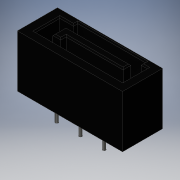
# Autodesk Inventor part: SATA_Conn_TH
Saved by Autodesk Inventor 2016 (Build 200138000, 138)
## iProperties
Created: 2017-03-04
Part Number: SATA_Conn_TH
Material: Generic
Document SubType Name: Modeling
Designer: jfixelle
Density: 1 g/cm^3
Appearance: Smooth - Black
Author: jfixelle
Autodesk Inventor part; units mm, degrees
ref_plane "YZ Plane" through (0, 0, 0) normal (1, 0, 0) x (0, 1, 0)
ref_plane "XZ Plane" through (0, 0, 0) normal (0, 1, 0) x (-1, 0, 0)
ref_plane "XY Plane" through (0, 0, 0) normal (0, 0, 1) x (1, 0, 0)
sketch "Sketch1" plane through (0, 0, 0) normal (0, 1, 0) x (-1, 0, 0)
  line L0 (8.45, 3.225) -> (-8.45, 3.225)
  line L1 (-8.45, 3.225) -> (-8.45, -3.225)
  line L2 (-8.45, -3.225) -> (8.45, -3.225)
  line L3 (8.45, -3.225) -> (8.45, 3.225)
  point P0 (0, 0)
  dimension "d0" = 16.9
  dimension "d1" = 8.45
  dimension "d2" = 6.45
  dimension "d3" = 3.225
  constraints: 8 end point, 2 parallel, 1 horizontal, 1 perpendicular
  measures "d0" distance of L1.end L2.end
  measures "d1" distance from line of point (0, 0) L3
  measures "d2" distance between parallel lines of L2 L0
  measures "d3" distance from line of point (0, 0) L2
extrude "Extrusion1" add sketch "Sketch1" along normal blind 8.4
sketch "Sketch2" plane through (0, 8.4, 0) normal (0, 1, 0) x (1, 0, 0)
  line L0 (-6.9642, -1.815) -> (7.0758, -1.815)
  line L1 (7.0758, -1.815) -> (7.0758, 2.125)
  line L2 (7.0758, 2.125) -> (-6.9642, 2.125)
  line L3 (-6.9642, 2.125) -> (-6.9642, -1.815)
  line L4 (6.0858, 2.125) -> (-4.7742, 2.125)
  line L5 (-4.7742, 2.125) -> (-4.7742, 2.825)
  line L6 (-4.7742, 2.825) -> (6.0858, 2.825)
  line L7 (6.0858, 2.825) -> (6.0858, 2.125)
  line L8 (-5.1242, -0.825) -> (-3.8742, -0.825)
  line L9 (-3.8742, -0.825) -> (-3.8742, 0.025)
  line L10 (-3.8742, 0.025) -> (5.2858, 0.025)
  line L11 (5.2858, 0.025) -> (5.2858, 1.275)
  line L12 (5.2858, 1.275) -> (-5.1242, 1.275)
  line L13 (-5.1242, 1.275) -> (-5.1242, -0.825)
  line L14 (-8.45, -3.225) -> (8.45, -3.225) projected
  point P0 (0, 0)
  dimension "d6" = 10.86
  dimension "d7" = 4.5
  dimension "d8" = 1.84
  dimension "d9" = 1.79
  dimension "d10" = 0.8
  dimension "d11" = 10.41
  dimension "d12" = 3.94
  dimension "d13" = 1.55
  dimension "d14" = 1.25
  dimension "d15" = 0.85
  dimension "d16" = 0.85
  dimension "d17" = 1.25
  constraints: 28 end point, 7 perpendicular, 4 parallel, 3 horizontal, 1 point on line
  measures "d6" distance of L5.end L6.end
  measures "d7" distance between parallel lines of L14 L12
  measures "d8" distance between parallel lines of L3 L13
  measures "d9" distance between parallel lines of L1 L11
  measures "d10" distance between parallel lines of L11 L7
  measures "d11" distance of L11.end L12.end
  measures "d12" distance between parallel lines of L2 L0
  measures "d13" distance between parallel lines of L6 L12
  measures "d14" distance between parallel lines of L12 L10
  measures "d15" distance between parallel lines of L4 L12
  measures "d16" distance between parallel lines of L10 L8
  measures "d17" distance of L8.start L8.end
extrude "Extrusion2" cut sketch "Sketch2" against normal blind 4.75
chamfer "Chamfer1" distance 0.2 angle 45 14 edges at (0.0808, 8.4, -1.275) (5.2858, 8.4, -0.65) (0.7058, 8.4, -0.025) (-3.8742, 8.4, 0.4) (-4.4992, 8.4, 0.825) (-5.1242, 8.4, -0.225) (-4.7742, 8.4, -2.475) (-5.8692, 8.4, -2.125) (-6.9642, 8.4, -0.155) (0.0558, 8.4, 1.815) (7.0758, 8.4, -0.155) (6.5808, 8.4, -2.125) (6.0858, 8.4, -2.475) (0.6558, 8.4, -2.825)
sketch "Sketch3" plane through (0, 0, 0) normal (0, -1, 0) x (1, 0, 0)
  line L0 (31.8884, 0.025) -> (-22.6507, 0.025) construction
  line L1 (42.8322, 1.525) -> (-5.5903, 1.525) construction
  circle A0 centre (0, 1.525) radius 0.225
  circle A1 centre (3.81, 1.525) radius 0.225
  circle A2 centre (-3.81, 1.525) radius 0.225
  circle A3 centre (-1.27, 0.025) radius 0.225
  circle A4 centre (-2.54, 0.025) radius 0.225
  circle A5 centre (1.27, 0.025) radius 0.225
  circle A6 centre (2.54, 0.025) radius 0.225
  line L2 (-4.9242, -1.075) -> (5.0858, -1.075) projected
  line L3 (4.5428, -1.075) -> (-4.5914, -1.075)
  point P0 (0, 0)
  dimension "d23" = 1.27
  dimension "d24" = 1.27
  dimension "d25" = 1.27
  dimension "d26" = 1.27
  dimension "d27" = 1.27
  dimension "d28" = 0
  dimension "d29" = 1.27
  dimension "d30" = 1.5
  dimension "d31" = 0.45
  dimension "d32" = 0.45
  dimension "d33" = 0.45
  dimension "d34" = 0.45
  dimension "d35" = 0.45
  dimension "d36" = 0.45
  dimension "d37" = 0.45
  dimension "d38" = 1.1
  constraints: 9 point on line, 7 centre point, 6 end point, 2 horizontal
  measures "d23" horizontal distance of A5.centre A0.centre
  measures "d24" distance of A6.centre A5.centre
  measures "d25" horizontal distance of A1.centre A6.centre
  measures "d26" horizontal distance of A3.centre A0.centre
  measures "d27" distance of A3.centre A4.centre
  measures "d28" horizontal distance of point (0, 0) A0.centre
  measures "d29" horizontal distance of A4.centre A2.centre
  measures "d30" distance between parallel lines of L1 L0
  measures "d31" diameter of A4
  measures "d32" diameter of A2
  measures "d33" diameter of A3
  measures "d34" diameter of A0
  measures "d35" diameter of A5
  measures "d36" diameter of A6
  measures "d37" diameter of A1
  measures "d38" distance between parallel lines of L0 L3
extrude "Extrusion3" add sketch "Sketch3" along normal blind 2.85
body "Solid1"
